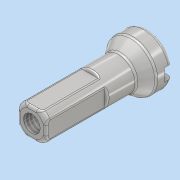
# Autodesk Inventor part: tornillo
Saved by Autodesk Inventor 2017 (Build 210142000, 142)
## iProperties
Part Number: tornillo
Material: Aluminio 6061
Document SubType Name: Modeling
Designer: Miguel A.
Density: 2.7 g/cm^3
Appearance: Aluminio - Pulido
Author: Miguel A.
Autodesk Inventor part; units mm, degrees
ref_plane "YZ Plane" through (0, 0, 0) normal (1, 0, 0) x (0, 1, 0)
ref_plane "XZ Plane" through (0, 0, 0) normal (0, 1, 0) x (-1, 0, 0)
ref_plane "XY Plane" through (0, 0, 0) normal (0, 0, 1) x (1, 0, 0)
sketch "Boceto1" plane through (0, 0, 0) normal (0, 0, 1) x (1, 0, 0)
  line L0 (0, 13.9855) -> (0, -13.9855)
  line L1 (0, 8.1846) -> (-3, 8.1846)
  line L2 (-3, 8.1846) -> (-3, 6.1846)
  line L3 (-3, 6.1846) -> (-2, 4.735)
  line L4 (-2, 4.735) -> (-2, -5.8154)
  line L5 (-2, -5.8154) -> (0, -5.8154)
  line L6 (0, -5.8154) -> (0, 8.1846)
  point P0 (0, 0)
  point P1 (0, 0)
  dimension "d0" = 6
  dimension "d1" = 4
  dimension "d2" = 34.6
  dimension "d3" = 2
  dimension "d4" = 14
  constraints: 14 end point, 2 point on line, 2 vertical, 1 coincident, 1 horizontal, 1 midpoint, 1 parallel, 1 perpendicular
  measures "d0" diameter of L2 L0
  measures "d1" diameter of L4 L0
  measures "d2" angle of L2 L3
  measures "d3" distance of L1.end L2.end
  measures "d4" distance between parallel lines of L1 L5
revolve "Revolución1" add sketch "Boceto1" angle 360 about axis through (0, 13.9855, 0) along (0, -1, 0)
fillet "Empalme1" radius 0.5 4 edges at (3, 8.1846, 0) (3, 6.1846, 0) (2, 4.735, 0) (2, -5.8154, 0)
hole "Agujero1" at (0, -5.8154, 0) direction (0, 1, 0) diameter 2.013 end through all thread size "M2.5x0.45" class "6H" standard "ISO Metric profile"
sketch "Boceto2" plane through (0, 8.1846, 0) normal (0, 1, 0) x (1, 0, 0)
  line L0 (-3.4183, -0.75) -> (4.0962, -0.75)
  line L1 (4.0962, -0.75) -> (4.0962, 0.75)
  line L2 (4.0962, 0.75) -> (-3.4183, 0.75)
  line L3 (-3.4183, 0.75) -> (-3.4183, -0.75)
  point P0 (0, 0)
  point P1 (-3.4183, 0)
  dimension "d18" = 1.5
  constraints: 8 end point, 2 parallel, 1 horizontal, 1 horizontal alignment, 1 midpoint, 1 perpendicular
  measures "d18" distance of L2.end L0.start
extrude "Extrusión1" cut sketch "Boceto2" against normal blind 1
sketch "Boceto3" plane through (0, -5.8154, 0) normal (0, -1, 0) x (1, 0, 0)
  line L0 (1.7, -1.7) -> (-1.7, -1.7)
  line L1 (-1.7, -1.7) -> (-1.7, 1.7)
  line L2 (-1.7, 1.7) -> (1.7, 1.7)
  line L3 (1.7, 1.7) -> (1.7, -1.7)
  circle A0 centre (0, 0) radius 2 construction
  circle A1 centre (0, 0) radius 2 construction
  line L4 (-3.9207, 3.8974) -> (3.9207, 3.8974)
  line L5 (3.9207, 3.8974) -> (3.9207, -3.8974)
  line L6 (3.9207, -3.8974) -> (-3.9207, -3.8974)
  line L7 (-3.9207, -3.8974) -> (-3.9207, 3.8974)
  circle A2 centre (0, 0) radius 1.5 projected
  line L8 (-3.9207, 3.8974) -> (3.9207, -3.8974) construction
  line L9 (3.9207, 3.8974) -> (-3.9207, -3.8974) construction
  point P0 (0, 0)
  point P1 (-1.7, 0)
  point P2 (0, -1.7)
  constraints: 20 end point, 4 midpoint, 4 parallel, 2 horizontal, 2 perpendicular, 1 horizontal alignment, 1 vertical alignment
extrude "Extrusión2" cut sketch "Boceto3" against normal blind 7 contours L4 L5 L6 L7
fillet "Empalme2" radius 0.3 18 edges at (0, -5.7736, 1.7) (1.0536, -2.0654, 1.7) (-1.0536, -2.0654, 1.7) (0, 1.1846, 2) (-1.7, -5.6696, -0.737) (-1.7, -5.6696, 0.737) (-1.7, -2.0654, -1.0536) (-1.7, -2.0654, 1.0536) (-1.9235, 1.1846, -0.5477) (-1.9235, 1.1846, 0.5477) (0, 1.1846, -2) (0, -5.7736, -1.7) (-1.0536, -2.0654, -1.7) (1.0536, -2.0654, -1.7) (1.7, -5.7736, 0) (1.7, -2.0654, 1.0536) (1.7, -2.0654, -1.0536) (2, 1.1846, 0)
ref_plane "Plano de trabajo1" through (0, 4.0846, 0) normal (0, 1, 0) x (1, 0, 0)
sketch "Boceto4" plane through (0, 4.0846, 0) normal (0, 1, 0) x (1, 0, 0)
  point P0 (0, 0)
  point P1 (0, 0)
  constraints: 1 coincident
